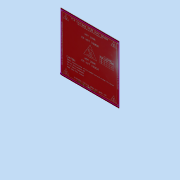
# Autodesk Inventor part: Part1
Saved by Autodesk Inventor 2015 (Build 190159000, 159)
## iProperties
Created: 2016-06-24
Part Number: Part1
Material: Generic
Document SubType Name: Modeling
Designer: Dustin
Density: 1 g/cm^3
Appearance: Default
Author: Dustin
Autodesk Inventor part; units mm, degrees
ref_plane "YZ Plane" through (0, 0, 0) normal (1, 0, 0) x (0, 1, 0)
ref_plane "XZ Plane" through (0, 0, 0) normal (0, 1, 0) x (-1, 0, 0)
ref_plane "XY Plane" through (0, 0, 0) normal (0, 0, 1) x (1, 0, 0)
sketch "Sketch3" plane through (0, 0, 0) normal (0, 0, 1) x (1, 0, 0)
  line L0 (0, 0) -> (214, 0)
  line L1 (214, 0) -> (214, 214)
  line L2 (214, 214) -> (0, 214)
  line L3 (0, 214) -> (0, 0)
  dimension "d2" = 214
  dimension "d3" = 214
  constraints: 8 end point, 2 parallel, 1 horizontal, 1 perpendicular
  measures "d2" distance of L0.start L0.end
  measures "d3" distance of L2.end L0.start
extrude "Extrusion1" add sketch "Sketch3" along normal blind 1.65
sketch "Sketch4" plane through (0, 0, 1.65) normal (0, 0, 1) x (1, 0, 0)
  line L0 (0.5008, 209.7083) -> (213.5162, 209.7083)
  line L1 (213.5162, 209.7083) -> (213.5162, 5.2135)
  line L2 (213.5162, 5.2135) -> (0.5008, 5.2135)
  line L3 (0.5008, 5.2135) -> (0.5008, 209.7083)
  constraints: 1 coincident, 2 other
body "Solid1"
